Spacer HS (Autodesk Fusion 360 design; units mm, degrees)
Autodesk Fusion 360 part; units mm, degrees
sketch "sketch 165" plane through (0, 0, 0) normal (1, 0, 0) x (0, -1, 0)
  circle A0 centre (0, 0) radius 5
  arc A1 (-2.1977, 3.2) -> (-2.2556, 3.1816) centre (-2.1977, 3.1) ccw
  arc A2 (2.2556, 3.1816) -> (2.1977, 3.2) centre (2.1977, 3.1) ccw
  line L0 (2.1977, 3.2) -> (-2.1977, 3.2)
  arc A3 (-3.1816, 2.2556) -> (-3.2, 2.1977) centre (-3.1, 2.1977) ccw
  arc A4 (3.2, 2.1977) -> (3.1816, 2.2556) centre (3.1, 2.1977) ccw
  arc A5 (3.1816, 2.2556) -> (2.2556, 3.1816) centre (0, 0) ccw
  arc A6 (-3.2, -2.1977) -> (-3.1816, -2.2556) centre (-3.1, -2.1977) ccw
  arc A7 (3.1816, -2.2556) -> (3.2, -2.1977) centre (3.1, -2.1977) ccw
  line L1 (3.2, -2.1977) -> (3.2, 2.1977)
  arc A8 (-2.2556, -3.1816) -> (-2.1977, -3.2) centre (-2.1977, -3.1) ccw
  arc A9 (-3.1816, -2.2556) -> (-2.2556, -3.1816) centre (0, 0) ccw
  arc A10 (2.1977, -3.2) -> (2.2556, -3.1816) centre (2.1977, -3.1) ccw
  arc A11 (2.2556, -3.1816) -> (3.1816, -2.2556) centre (0, 0) ccw
  line L2 (-2.1977, -3.2) -> (2.1977, -3.2)
  line L3 (-3.2, 2.1977) -> (-3.2, -2.1977)
  arc A12 (-2.2556, 3.1816) -> (-3.1816, 2.2556) centre (0, 0) ccw
extrude "Extrude1" add sketch "sketch 165" along normal blind 1.5875
fillet "Fillet1" radius 0.254 2 faces at (1.5875, 3.8, 0) (0, 3.8, 0)
